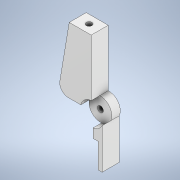
# Autodesk Inventor part: pliers
Saved by Autodesk Inventor 2020 (Build 240168000, 168)
## iProperties
Created: 2019-12-24
Part Number: pliers
Material: ABS Plastic
Document SubType Name: Modeling
Designer: metal
Density: 1.06 g/cm^3
Appearance: Smooth - White
Author: metal
Autodesk Inventor part; units mm, degrees
ref_plane "YZ Plane" through (0, 0, 0) normal (1, 0, 0) x (0, 1, 0)
ref_plane "XZ Plane" through (0, 0, 0) normal (0, 1, 0) x (-1, 0, 0)
ref_plane "XY Plane" through (0, 0, 0) normal (0, 0, 1) x (1, 0, 0)
sketch "Sketch1" plane through (0, 0, 0) normal (0, 0, 1) x (1, 0, 0)
  circle A0 centre (0, 0) radius 4
  line L0 (0, 24) -> (-8, 24)
  line L1 (0, 24) -> (0, 4)
  line L2 (-11.9043, 0.8695) -> (-3.9043, 0.8695)
  line L3 (-11.9043, 0.8695) -> (-8, 24)
  dimension "d9" = 6
  dimension "d0" = 8
  dimension "d6" = 8
  dimension "d94" = 20
  dimension "d95" = 8
  constraints: 8 end point, 2 horizontal, 2 point on circle, 1 centre point, 1 coincident, 1 vertical
  measures "d0" diameter of A0
  measures "d6" distance of L0.start L0.end
  measures "d94" distance of L0.start L1.end
  measures "d95" distance of L2.start L2.end
extrude "Extrusion1" add sketch "Sketch1" along normal mid plane 6
sketch "Sketch2" plane through (0, 0, 3) normal (0, 0, 1) x (1, 0, 0)
  circle A0 centre (0, 0) radius 4
  constraints: 1 centre point, 1 coincident
extrude "Extrusion2" cut sketch "Sketch2" against normal blind 3
sketch "Sketch4" plane through (-8, 24, 3) normal (0, 1, 0) x (1, 0, 0)
  line L0 (8, 6) -> (8, 0) projected
  line L1 (0, 0) -> (8, 6)
  line L2 (8, 0) -> (0, 0) projected
  line L3 (0, 6) -> (0, 0) projected
  line L4 (8, 0) -> (0, 6)
  circle A0 centre (4, 3) radius 1
  point P0 (8, 3)
  point P1 (3.2, 2.4)
  point P2 (3.2, 3.6)
  dimension "d9" = 6
  dimension "d17" = 2
  dimension "d93" = 1.2
  constraints: 4 end point, 2 point on circle, 1 centre point, 1 midpoint
  measures "d17" diameter of A0
  measures "d93" distance of A0.start A0.end
extrude "Extrusion4" cut sketch "Sketch4" against normal blind 5 contours A0 L4 L1 | L1 L4 A0 | A0 L1 L4 | L1 A0 L4
sketch "Sketch8" plane through (0, 0, 0) normal (0, 0, 1) x (1, 0, 0)
  arc A0 (-3.9043, 0.8695) -> (0, 4) centre (0, 0) ccw projected
  dimension "d9" = 6
  constraints: 1 coincident
hole "Hole3" at (0, 0, 0) direction (0, 0, -1) diameter 2.1 end through all
sketch "Sketch9" plane through (0, 0, 0) normal (0, 0, 1) x (1, 0, 0)
  line L0 (0, 4) -> (0, 24) construction
  line L1 (0, 24) -> (-8, 24) construction
  line L2 (-3.2679, 22.7321) -> (-9.3121, 0.175) construction
  line L3 (-11.9043, 0.8695) -> (-3.9043, 0.8695) construction
  arc A0 (0, 4) -> (-3.9043, 0.8695) centre (0, 0) ccw construction
  arc A1 (-3.9043, 0.8695) -> (0, 4) centre (0, 0) ccw projected
  line L4 (0, 31.995) -> (0, -23.9701) construction
  arc A2 (-3.9043, 0.8695) -> (0, 4) centre (0, 0) ccw construction
  line L5 (0.446, -3.9751) -> (0.446, -10.9751)
  line L6 (3.846, -1.0991) -> (3.846, -15.9751)
  line L7 (0.446, -10.9751) -> (2.246, -10.9751)
  line L8 (2.246, -10.9751) -> (2.246, -15.9751)
  line L9 (2.246, -15.9751) -> (3.846, -15.9751)
  point P0 (0.446, -3.9751)
  dimension "d9" = 6
  dimension "d90" = 7
  dimension "d91" = 3.4
  dimension "d92" = 1.8
  constraints: 10 end point, 2 perpendicular, 2 point on circle, 2 vertical, 1 horizontal
  measures "d90" distance of L5.start L5.end
  measures "d91" horizontal distance of L6.start L5.start
  measures "d92" distance of L5.end L7.end
extrude "Extrusion5" add sketch "Sketch9" along normal mid plane 6
sketch "Sketch10" plane through (0, 0, -3) normal (0, 0, -1) x (-1, 0, 0)
  circle A0 centre (0, 0) radius 1.05 projected
  circle A1 centre (0, 0) radius 1.8
  dimension "d9" = 6
  dimension "d62" = 3.6
  constraints: 1 centre point, 1 coincident
  measures "d62" diameter of A1
extrude "Extrusion6" cut sketch "Sketch10" against normal blind 1
fillet "Fillet2" radius 3 1 edges at (-11.9043, 0.8695, 0)
move faces "Move1" translate (-0.25, 0, 0) faces at (3.846, -11.0164, 0)
move faces "Move2" translate (-0.25, 0, 0) faces at (0, 17.3333, 0)
move faces "Move3" translate (0, 3.75, 0) faces at (1.646, -10.9751, 1)
body "Solid1"
